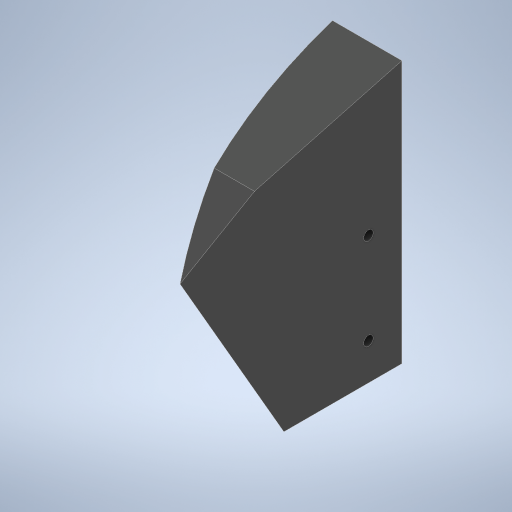
# Autodesk Inventor part: chest_base_left
Saved by Autodesk Inventor 2024.1 (Build 281209000, 209)
## iProperties
Created: 2024-10-10
Part Number: chest_base_left
Material: 一般
Document SubType Name: Modeling
Designer: hibik
Density: 1 g/cm^3
Appearance: 既定
Author: hibik
Autodesk Inventor part; units mm, degrees
ref_plane "YZ Plane" through (0, 0, 0) normal (1, 0, 0) x (0, 1, 0)
ref_plane "XZ Plane" through (0, 0, 0) normal (0, 1, 0) x (-1, 0, 0)
ref_plane "XY Plane" through (0, 0, 0) normal (0, 0, 1) x (1, 0, 0)
sketch "スケッチ1" plane through (0, 0, 0) normal (1, 0, 0) x (0, 1, 0)
  line L0 (0, 0) -> (27, 0)
  line L1 (27, 0) -> (27, 35)
  line L2 (27, 35) -> (0, 35)
  line L3 (0, 35) -> (0, 0)
  line L4 (27, 35) -> (0, 19.4115)
  arc A0 (47.2073, 0) -> (27, 35) centre (6.7927, 0) ccw construction
  line L5 (47.2073, 0) -> (47.2073, 12.8727) construction
  line L6 (27, 0) -> (47.2073, 0)
  circle A1 centre (21, 5.5) radius 0.8
  circle A2 centre (6, 5.5) radius 0.8
  line L7 (27, 35) -> (29.5981, 36.5)
  line L8 (47.2073, 0) -> (51.2073, 0)
  line L9 (27, 35) -> (47.2073, 0) construction
  line L10 (29.5981, 36.5) -> (50.6714, 0)
  dimension "d0" = 27
  dimension "d1" = 35
  dimension "d2" = 30
  dimension "d7" = 1.6
  dimension "d8" = 5.5
  dimension "d9" = 6
  dimension "d10" = 6
  dimension "d20" = 30
  dimension "d24" = 3
  constraints: 22 end point, 3 centre point, 3 horizontal, 3 horizontal alignment, 3 parallel, 2 point on circle, 2 point on line, 1 collinear, 1 equal radius, 1 perpendicular, 1 tangent, 1 vertical
  measures "d0" distance of L2.end L1.end
  measures "d1" distance of L1.end L0.end
  measures "d2" angle of L2 L4
  measures "d7" diameter of A1
  measures "d8" distance from line of L0 A1.centre
  measures "d9" distance from line of L1 A1.centre
  measures "d10" distance from line of L3 A2.centre
  measures "d20" angle of L1 L9
  measures "d24" distance between parallel lines of L9 L10
extrude "押し出し1" add sketch "スケッチ1" along normal blind 11.5 contours L3 L4 L1 L0 | L1 L7 L10 L8 L6
sketch "スケッチ7" plane through (0, 29.5981, 36.5) normal (0, 0.8660254, 0.5) x (1, 0, 0)
  line L0 (11.5, 16.8109) -> (11.5, 42.1466) projected
  arc A0 (0, 0) -> (11.5, 42.1466) centre (-71.4819, 42.1466) ccw
  line L1 (11.5, 42.1466) -> (11.5, 0) projected
  line L2 (0, 0) -> (11.5, 0) projected
  point P0 (0, 16.8109)
  constraints: 2 point on circle, 1 centre point, 1 tangent
extrude "押し出し5" cut sketch "スケッチ7" against normal through all
sketch "スケッチ8" plane through (0, 0, 0) normal (-1, 0, 0) x (0, 0, 1)
  line L0 (0, 0) -> (8, 3)
  line L1 (8, 3) -> (8, 24)
  line L2 (8, 24) -> (0, 27)
  circle A0 centre (5.5, 21) radius 0.8 projected
  line L3 (0, 0) -> (0, 50.6714) projected
  circle A1 centre (5.5, 6) radius 0.8 projected
  dimension "d28" = 3
  dimension "d29" = 3
  dimension "d30" = 8
  dimension "d31" = 3
  constraints: 6 end point, 1 point on line, 1 vertical
  measures "d28" vertical distance of L0.start L0.end
  measures "d29" vertical distance of L1.end A0.centre
  measures "d30" distance between parallel lines of L3 L1
  measures "d31" vertical distance of L1.end L2.end
extrude "押し出し6" add sketch "スケッチ8" against normal up to surface (11.5 mm away)
sketch "スケッチ9" plane through (0, 0, 0) normal (-1, 0, 0) x (0, 0, 1)
  line L0 (0, 50.6714) -> (36.5, 29.5981) projected
  line L1 (0, 0) -> (0, 50.6714) projected
  line L2 (0, 43.1688) -> (24.2487, 36.6714)
  dimension "d37" = 14
  dimension "d38" = 15
  constraints: 2 end point, 2 point on line
  measures "d37" vertical distance of L0.start L2.end
  measures "d38" angle of L0 L2
extrude "押し出し7" cut sketch "スケッチ9" against normal through all
mirror "ミラー1" about plane through (0, 13.5, 17.5) normal (-1, 0, 0) remove original yes
equation "\"d10\" = d9"
equation "\"d29\" = d28"
